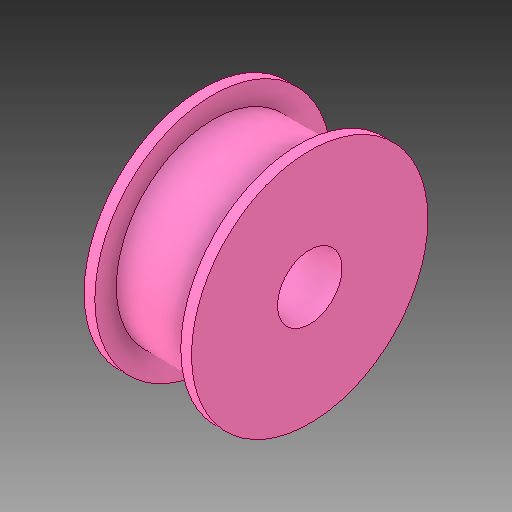
# Autodesk Inventor part: pulley XL 1.25in
Saved by Autodesk Inventor 2017 SP1 (Build 210196100, 196)
## iProperties
Created: 2018-01-21
Part Number: pulley XL 1.25in
Material: Nylon 6/6
Document SubType Name: Modeling
Designer: Ben
Density: 1.13 g/cm^3
Appearance: Pink
Mass: 11.3621 g
Surface Area: 43.7035 cm^2
Volume: 10.055 cm^3
Author: Ben
Autodesk Inventor part; units mm, degrees
ref_plane "YZ Plane" through (0, 0, 0) normal (1, 0, 0) x (0, 1, 0)
ref_plane "XZ Plane" through (0, 0, 0) normal (0, 1, 0) x (-1, 0, 0)
ref_plane "XY Plane" through (0, 0, 0) normal (0, 0, 1) x (1, 0, 0)
sketch "Sketch1" plane through (0, 0, 0) normal (1, 0, 0) x (0, 1, 0)
  circle A0 centre (0, 0) radius 14.2875
  circle A1 centre (0, 0) radius 4.7625
  dimension "d0" = 28.575
  dimension "d2" = 9.525
  constraints: 2 centre point, 2 coincident
  measures "d0" diameter of A0
  measures "d2" diameter of A1
extrude "Extrusion1" add sketch "Sketch1" along normal mid plane 12.7
sketch "Sketch2" plane through (6.35, 0, 0) normal (1, 0, 0) x (0, 0, -1)
  circle A0 centre (0, 0) radius 17.4625
  circle A1 centre (0, 0) radius 14.2875 construction
  circle A2 centre (0, 0) radius 4.7625 projected
  dimension "d6" = 3.175
  constraints: 1 centre point, 1 coincident
  measures "d6" radial gap between concentric circles of A1 A0
extrude "Extrusion2" add sketch "Sketch2" along normal blind 1.5875
sketch "Sketch3" plane through (-6.35, 0, 0) normal (-1, 0, 0) x (0, 0, 1)
  circle A0 centre (0, 0) radius 17.4625 projected
  circle A1 centre (0, 0) radius 4.7625 projected
extrude "Extrusion3" add sketch "Sketch3" along normal blind 1.5875
sketch "Sketch4" plane through (7.9375, 0, 0) normal (1, 0, 0) x (0, 0, -1)
  circle A0 centre (0, 0) radius 4.7625 projected
  circle A1 centre (0, 0) radius 9.525
  dimension "d11" = 4.7625
  constraints: 1 centre point, 1 coincident
  measures "d11" radial gap between concentric circles of A0 A1
extrude "Extrusion4" [suppressed]
body "Solid1"
